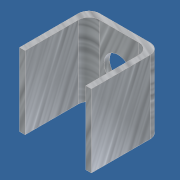
# Autodesk Inventor part: 2009_CTS_UClip
Saved by Autodesk Inventor 2012 (Build 160160000, 160)
## iProperties
Company: Team 801
Created: 2009-01-31
Part Number: 2009_CTS_UClip
Material: Aluminum-6061
Document SubType Name: Modeling
Designer: Jeffrey M
Mass: 0.301398 g
Surface Area: 3.67377 cm^2
Volume: 0.111217 cm^3
Density: 2.71 g/cm^3
Title: 2009_CTS_UClip
Author: Jeffrey M
Autodesk Inventor part; units mm, degrees
ref_plane "YZ Plane" through (0, 0, 0) normal (1, 0, 0) x (0, 1, 0)
ref_plane "XZ Plane" through (0, 0, 0) normal (0, 1, 0) x (-1, 0, 0)
ref_plane "XY Plane" through (0, 0, 0) normal (0, 0, 1) x (1, 0, 0)
sketch "Sketch1" plane through (0, 0, 0) normal (0, 0, 1) x (1, 0, 0)
  line L0 (-4.4793, 2.7495) -> (-12.9883, 2.7495)
  line L1 (-12.9883, 2.7495) -> (-12.9883, 11.3855)
  line L2 (-12.9883, 11.3855) -> (-4.4793, 11.3855)
  line L3 (-4.4793, 11.3855) -> (-4.4793, 2.7495)
  dimension "d0" = 8.509
  dimension "d1" = 8.636
  constraints: 8 end point, 2 parallel, 1 horizontal, 1 perpendicular
  measures "d0" distance of L1.end L2.end
  measures "d1" distance of L2.end L0.start
extrude "Extrusion1" add sketch "Sketch1" along normal blind 0.6604
sketch "Sketch2" plane through (0, 0, 0.6604) normal (0, 0, 1) x (1, 0, 0)
  line L0 (-12.9883, 2.7495) -> (-12.9883, 11.3855) projected
  line L1 (-4.4793, 2.7495) -> (-12.9883, 2.7495) projected
  line L2 (-4.4793, 11.3855) -> (-4.4793, 2.7495) projected
  line L3 (-12.9883, 11.3855) -> (-12.3279, 11.3855)
  line L4 (-12.3279, 11.3855) -> (-12.3279, 2.7495)
  line L5 (-12.3279, 2.7495) -> (-12.9883, 2.7495)
  line L6 (-12.9883, 2.7495) -> (-12.9883, 11.3855)
  line L7 (-4.4793, 11.3855) -> (-5.1397, 11.3855)
  line L8 (-5.1397, 11.3855) -> (-5.1397, 2.7495)
  line L9 (-5.1397, 2.7495) -> (-4.4793, 2.7495)
  line L10 (-4.4793, 2.7495) -> (-4.4793, 11.3855)
  dimension "d4" = 0.6604
  dimension "d5" = 0.6604
  constraints: 16 end point, 4 parallel, 2 horizontal, 2 perpendicular, 2 point on line
  measures "d4" distance of L0.end L3.end
  measures "d5" distance between parallel lines of L2 L8
extrude "Extrusion2" add sketch "Sketch2" along normal blind 7.5692
fillet "Fillet1" radius 1.27 2 edges at (-4.4793, 7.0675, 0) (-12.9883, 7.0675, 0)
fillet "Fillet2" radius 1.27 2 edges at (-12.3279, 7.0675, 0.6604) (-5.1397, 7.0675, 0.6604)
sketch "Sketch3" plane through (0, 0, 0) normal (0, 0, -1) x (-1, 0, 0)
  point P0 (8.8865, 7.2342)
hole "Hole1" at (-8.8865, 7.2342, 0) direction (0, 0, 1) diameter 3.3274 depth 19.05 tip angle 118
sketch "Sketch4" plane through (0, 0, 0) normal (0, 0, -1) x (-1, 0, 0)
  circle A0 centre (8.8865, 7.2342) radius 1.6637 projected
body "Solid1"
